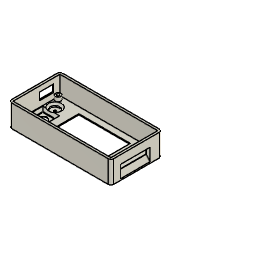
Display Mount - TFT24V1_1 Cover SD Access (Autodesk Fusion 360 design; units mm, degrees)
Autodesk Fusion 360 part; units mm, degrees
note: some values were not read from the file. Set by a fixed rule: which sketch regions a step uses.
sketch "Sketch1" plane through (0, 0, -2.4) normal (0, 0, 1) x (-1, 0, 0)
  line L0 (-47.615, 23) -> (47.58, 23)
  line L1 (47.58, 23) -> (47.58, -23)
  line L2 (47.58, -23) -> (-47.615, -23)
  line L3 (-47.615, -23) -> (-47.615, 23)
  circle A0 centre (50.04, 20.575) radius 1.75
  circle A1 centre (50.04, -20.575) radius 1.75
  circle A2 centre (-50.04, -20.575) radius 1.75
  circle A3 centre (-50.04, 20.575) radius 1.75
  line L4 (52.5, -22) -> (52.5, 22)
  line L5 (49.5, 25) -> (-49.5, 25)
  line L6 (-52.5, 22) -> (-52.5, -22)
  line L7 (-49.5, -25) -> (49.5, -25)
  line L8 (52.7, 25.2) -> (-52.7, 25.2)
  line L9 (-52.7, 25.2) -> (-52.7, -25.2)
  line L10 (-52.7, -25.2) -> (52.7, -25.2)
  line L11 (52.7, -25.2) -> (52.7, 25.2)
  line L12 (55.1, 27.6) -> (-55.1, 27.6)
  line L13 (-55.1, 27.6) -> (-55.1, -27.6)
  line L14 (-55.1, -27.6) -> (55.1, -27.6)
  line L15 (55.1, -27.6) -> (55.1, 27.6)
  arc A4 (-52.5, -22) -> (-49.5, -25) centre (-49.5, -22) ccw
  arc A5 (49.5, -25) -> (52.5, -22) centre (49.5, -22) ccw
  arc A6 (52.5, 22) -> (49.5, 25) centre (49.5, 22) ccw
  arc A7 (-49.5, 25) -> (-52.5, 22) centre (-49.5, 22) ccw
  constraint parallel L5 L8
  constraint parallel L6 L9
  constraint parallel L7 L10
  constraint parallel L4 L11
  constraint parallel L5 L12
  constraint parallel L6 L13
  constraint parallel L7 L14
  constraint parallel L4 L15
extrude "Extrude1" add sketch "Sketch1" against normal blind 20 contours L12 L13 L14 L15
sketch "Sketch2" plane through (0, 0, -22.4) normal (0, 0, -1) x (1, 0, 0)
  line L0 (-52.7, -25.2) -> (-52.7, 25.2)
  line L1 (-52.7, 25.2) -> (52.7, 25.2)
  line L2 (52.7, 25.2) -> (52.7, -25.2)
  line L3 (52.7, -25.2) -> (-52.7, -25.2)
  line L4 (-55.1, 27.6) -> (-55.1, -27.6)
  line L5 (-55.1, -27.6) -> (55.1, -27.6)
  line L6 (55.1, -27.6) -> (55.1, 27.6)
  line L7 (55.1, 27.6) -> (-55.1, 27.6)
extrude "Extrude2" add sketch "Sketch2" along normal blind 4 contours L0 L1 L2 L3 | L4 L5 L6 L7
sketch "Sketch3" plane through (0, 0, -26.4) normal (0, 0, -1) x (1, 0, 0)
  line L0 (-55.1, 27.6) -> (-55.1, -27.6)
  line L1 (0, 49.8333) -> (0, -49.8333) construction
  line L2 (-25.55, 20.25) -> (29.8, 20.25)
  line L3 (29.8, 20.25) -> (29.8, -18.5)
  line L4 (29.8, -18.5) -> (-25.55, -18.5)
  line L5 (-25.55, -18.5) -> (-25.55, 20.25)
  line L6 (-52.55, 25) -> (52.55, 25)
  line L7 (52.55, 25) -> (52.55, -21) construction
  line L8 (52.55, -21) -> (-52.55, -21) construction
  line L9 (-52.55, -21) -> (-52.55, 25) construction
  line L10 (55.1, -27.6) -> (55.1, 27.6)
  line L11 (-55.1, -27.6) -> (55.1, -27.6)
  line L12 (55.1, 27.6) -> (-55.1, 27.6)
  circle A0 centre (-44.55, -11.8) radius 5
  circle A1 centre (-44.55, -11.8) radius 1
  circle A2 centre (-43.05, 2.8) radius 4.3
  line L13 (-36.55, -3.7) -> (-49.55, -3.7)
  line L14 (-49.55, -3.7) -> (-49.55, 9.3)
  line L15 (-49.55, 9.3) -> (-36.55, 9.3)
  line L16 (-36.55, 9.3) -> (-36.55, -3.7)
  line L17 (-49.55, -3.7) -> (-36.55, 9.3) construction
  circle A3 centre (-38.95, 19.5) radius 2.3
  point P0 (-43.05, 2.8)
  point P1 (0, -21)
  point P2 (52.55, 2)
  dimension "d137" = 4.75
  dimension "d138" = 27
  dimension "d139" = 22.75
  dimension "d140" = 2.5
  dimension "d141" = 54.9
  dimension "d142" = 42.95
  dimension "d143" = 10
  dimension "d144" = 2
  dimension "d145" = 9.2
  dimension "d146" = 8
  dimension "d147" = 8.6
  dimension "d148" = 23.8
  dimension "d149" = 9.5
  dimension "d150" = 13
  dimension "d151" = 13
  dimension "d152" = 4.6
  dimension "d153" = 13.6
  dimension "d154" = 5.5
  dimension "d174" = 46
  dimension "d175" = 105.1
  dimension "d207" = 2.6
  constraint midpoint origin L1
  constraint horizontal L2
  constraint horizontal L4
  constraint vertical L5
  constraint horizontal L6
  constraint vertical L7
  constraint horizontal L8
  constraint vertical L9
  constraint concentric A0 A1
  constraint horizontal L13
  constraint vertical L14
  constraint horizontal L15
  constraint vertical L16
  constraint midpoint L17 P0
  constraint coincident P0 A2.centre
  constraint midpoint L8 P1
  constraint midpoint L7 P2
  constraint vertical origin P1
  measures "d137" distance of L2 L6
  measures "d138" distance of L5 L9
  measures "d139" distance of L3 L7
  measures "d140" distance of L4 L8
  measures "d143" diameter of A0
  measures "d144" diameter of A1
  measures "d145" distance of L8 A0.centre
  measures "d146" distance of L9 A0.centre
  measures "d147" diameter of A2
  measures "d148" distance of L8 P0
  measures "d149" distance of L9 P0
  measures "d150" distance of L13.start L13.end
  measures "d151" distance of L13.start L15.end
  measures "d152" diameter of A3
  measures "d153" distance of L9 A3.centre
  measures "d154" distance of L6 A3.centre
  measures "d174" distance of L6.end L7.end
  measures "d175" distance of L7.end L8.end
  measures "d207" distance of L6 L12
extrude "Extrude14" cut sketch "Sketch3" against normal blind 4 from surface at -0.6 contours L13 L14 L15 L16
extrude "Extrude15" cut sketch "Sketch3" against normal blind 4 from surface at -0.6 contours A0
extrude "Extrude12" cut sketch "Sketch3" against normal blind 4 contours A3
extrude "Extrude11" cut sketch "Sketch3" against normal blind 4 contours A2
extrude "Extrude10" cut sketch "Sketch3" against normal blind 4 contours A1
extrude "Extrude7" cut sketch "Sketch3" against normal blind 4 contours L2 L3 L4 L5
chamfer "Chamfer9" distance 2.5 angle 45 4 edges at (-43.05, 3.7, -22.4) (-49.55, -2.8, -22.4) (-43.05, -9.3, -22.4) (-36.55, -2.8, -22.4)
chamfer "Chamfer8" distance 2 angle 45 1 edges at (-49.2116, 13.6081, -22.4)
chamfer "Chamfer1" distance 3 angle 45 4 edges at (2.125, -20.25, -26.4) (-25.55, -0.875, -26.4) (29.8, -0.875, -26.4) (2.125, 18.5, -26.4)
sketch "Sketch5" plane through (-55.1, 0, 0) normal (-1, 0, 0) x (0, -1, 0)
  line L0 (27.6, -2.4) -> (-27.6, -2.4)
  line L1 (-27.6, -2.4) -> (-27.6, -20)
  line L2 (-27.6, -20) -> (27.6, -20)
  line L3 (27.6, -20) -> (27.6, -2.4)
  line L4 (-5, -8.4) -> (-5, -16.4)
  line L5 (-18.4, -8.1) -> (-3.4, -8.1)
  line L6 (-3.4, -8.1) -> (-3.4, -16.1)
  line L7 (-3.4, -16.1) -> (-18.4, -16.1)
  line L8 (-18.4, -16.1) -> (-18.4, -8.1)
  line L9 (27.6, -2.4) -> (-27.6, -2.4)
  line L10 (-27.6, -2.4) -> (-27.6, -26.4)
  line L11 (-27.6, -26.4) -> (27.6, -26.4)
  line L12 (27.6, -26.4) -> (27.6, -2.4)
  line L13 (27.6, -26.4) -> (-27.6, -26.4)
  line L14 (-20.4, -6.1) -> (-1.4, -6.1)
  line L15 (-1.4, -6.1) -> (-1.4, -18.1)
  line L16 (-1.4, -18.1) -> (-20.4, -18.1)
  line L17 (-20.4, -18.1) -> (-20.4, -6.1)
  dimension "d107" = 15
  dimension "d108" = 8
  dimension "d109" = 9.2
  dimension "d191" = 10.3
  dimension "d193" = -2
  constraint horizontal L5
  constraint vertical L6
  constraint horizontal L7
  constraint vertical L8
  measures "d107" distance of L5.start L5.end
  measures "d108" distance of L5 L7
  measures "d109" distance of L1 L8
  measures "d191" distance of L7 L13
extrude "Extrude16" cut sketch "Sketch5" against normal blind 1 contours L14 L15 L16 L17
extrude "Extrude8" cut sketch "Sketch5" against normal blind 3 contours L5 L6 L7 L8
sketch "Sketch6" plane through (55.1, 0, 0) normal (1, 0, 0) x (0, 1, 0)
  line L0 (28.2, -2.4) -> (-28.2, -2.4)
  line L1 (-28.2, -2.4) -> (-28.2, -20)
  line L2 (-28.2, -20) -> (28.2, -20)
  line L3 (28.2, -20) -> (28.2, -2.4)
  line L4 (-15, -13.4) -> (-15, -16.4)
  line L5 (12.5, -13.4) -> (-15, -13.4)
  line L6 (12.5, -16.4) -> (12.5, -13.4)
  line L7 (12.5, -17.85) -> (-15, -17.85)
  line L8 (-15, -17.85) -> (-15, -13.25)
  line L9 (-15, -13.25) -> (12.5, -13.25)
  line L10 (12.5, -13.25) -> (12.5, -17.85)
  line L11 (28.2, -20) -> (-28.2, -20)
  line L12 (27.6, -2.4) -> (-27.6, -2.4)
  line L13 (-27.6, -2.4) -> (-27.6, -26.4)
  line L14 (-27.6, -26.4) -> (27.6, -26.4)
  line L15 (27.6, -26.4) -> (27.6, -2.4)
  point P0 (-15, -15.55)
  dimension "d118" = 27.5
  dimension "d119" = 15.7
  dimension "d120" = 4.6
  dimension "d210" = 10.85
  constraint horizontal L7
  constraint vertical L8
  constraint vertical L10
  constraint coincident L9.end L10.start
  constraint perpendicular L9 L10
  constraint midpoint L8 P0
  measures "d118" distance of L8 L10
  measures "d119" distance of L3 L10
  measures "d120" distance of L7 L9
  measures "d210" distance of L14 P0
extrude "Extrude18" cut sketch "Sketch6" against normal blind 2.4 contours L4 L5 L6 L7 L8 L10
fillet "Fillet1" radius 3 4 edges at (55.1, 27.6, -14.4) (55.1, -27.6, -14.4) (-55.1, -27.6, -14.4) (-55.1, 27.6, -14.4)
chamfer "Chamfer14" distance 1 angle 45 4 edges at (-55.1, 20.4, -12.1) (-55.1, 10.9, -6.1) (-55.1, 1.4, -12.1) (-55.1, 10.9, -18.1)
sketch "Sketch7" plane through (0, 0, -22.4) normal (0, 0, 1) x (-1, 0, 0)
  arc A0 (40.35, -6.2) -> (48.75, -6.2) centre (44.55, -11.8) ccw
  line L0 (40.35, -6.2) -> (34.05, -6.2)
  line L1 (34.05, -6.2) -> (34.05, 11.8)
  line L2 (34.05, 11.8) -> (52.05, 11.8)
  line L3 (52.05, 11.8) -> (52.05, -6.2)
  line L4 (52.05, -6.2) -> (48.75, -6.2)
  line L5 (-52.7, -25.2) -> (52.7, -25.2)
  line L6 (52.7, -25.2) -> (52.7, 25.2)
  line L7 (52.7, 25.2) -> (-52.7, 25.2)
  line L8 (-52.7, 25.2) -> (-52.7, -25.2)
  circle A1 centre (38.95, 19.5) radius 2.3
  line L9 (-29.8, -18.5) -> (-29.8, 20.25)
  line L10 (-29.8, 20.25) -> (25.55, 20.25)
  line L11 (25.55, 20.25) -> (25.55, -18.5)
  line L12 (25.55, -18.5) -> (-29.8, -18.5)
  circle A2 centre (-50.04, -20.575) radius 1.75
  circle A3 centre (-50.04, -20.575) radius 1.75
  circle A4 centre (-50.04, 20.575) radius 1.75
  circle A5 centre (50.04, 20.575) radius 1.75
  circle A6 centre (50.04, -20.575) radius 1.75
  circle A7 centre (50.04, 20.575) radius 1.425
  circle A8 centre (50.04, -20.575) radius 1.425
  circle A9 centre (-50.04, -20.575) radius 1.425
  circle A10 centre (-50.04, 20.575) radius 1.425
  circle A11 centre (50.04, -20.575) radius 3
  circle A12 centre (50.04, 20.575) radius 3
  circle A13 centre (-50.04, -20.575) radius 3
  circle A14 centre (-50.04, 20.575) radius 3
  arc A15 (48.3872, -20) -> (51.6928, -20) centre (50.04, -20.575) ccw
  dimension "d197" = 2.85
  dimension "d198" = 2.85
  dimension "d199" = 2.85
  dimension "d200" = 2.85
  dimension "d216" = 6
  dimension "d217" = 6
  dimension "d218" = 6
  dimension "d219" = 6
  constraint concentric A5 A7
  constraint concentric A6 A8
  constraint concentric A2 A9
  constraint concentric A4 A10
  constraint concentric A6 A11
  constraint concentric A5 A12
  constraint concentric A2 A13
  constraint concentric A4 A14
  measures "d197" diameter of A7
  measures "d198" diameter of A8
  measures "d199" diameter of A9
  measures "d200" diameter of A10
  measures "d216" diameter of A11
  measures "d217" diameter of A13
  measures "d218" diameter of A12
  measures "d219" diameter of A14
extrude "Extrude19" add sketch "Sketch7" along normal blind 4.4 contours L8 A13 | L6 A11 | L8 A14 | L6 A12 | A2 A3 | A4 | A5 | A6 A15 picked at (-52.3967, -20.575) picked at (52.3967, -20.575) picked at (-52.3967, 20.575) picked at (52.3967, 20.575)
extrude "Extrude17" cut sketch "Sketch7" against normal blind 3.6 contours A7 | A8 | A9 | A10
chamfer "Chamfer16" distance 2 angle 45 3 edges at (55.1, 12.5, -15.625) (55.1, -1.25, -13.4) (55.1, -15, -15.625)
chamfer "Chamfer17" distance 7 distance2 2 1 edges at (55.1, -1.25, -17.85) measured on face at (55.1, 21.2333, -13.4)
equation "d169 = 0 mm - 0.600 mm"
equation "d217 = d216"
equation "d218 = d216"
equation "d219 = d216"
